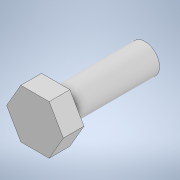
# Autodesk Inventor part: M4_short
Saved by Autodesk Inventor 2022 (Build 260153000, 153)
## iProperties
Created: 2022-02-22
Part Number: M4_short
Material: Generic
Document SubType Name: Modeling
Designer: katha
Density: 1 g/cm^3
Appearance: Default
Author: katha
Autodesk Inventor part; units mm, degrees
ref_plane "YZ Plane" through (0, 0, 0) normal (1, 0, 0) x (0, 1, 0)
ref_plane "XZ Plane" through (0, 0, 0) normal (0, 1, 0) x (-1, 0, 0)
ref_plane "XY Plane" through (0, 0, 0) normal (0, 0, 1) x (1, 0, 0)
sketch "Sketch1" plane through (0, 0, 0) normal (0, 0, 1) x (1, 0, 0)
  line L0 (0, 0) -> (3.9, 0) construction
  line L1 (0, 0) -> (1.95, 3.3775) construction
  line L2 (0, 0) -> (-1.95, 3.3775) construction
  line L3 (0, 0) -> (-3.9, 0) construction
  line L4 (0, 0) -> (-1.95, -3.3775) construction
  line L5 (0, 0) -> (1.95, -3.3775) construction
  line L6 (-1.95, 3.3775) -> (1.95, 3.3775)
  line L7 (1.95, 3.3775) -> (3.9, 0)
  line L8 (3.9, 0) -> (1.95, -3.3775)
  line L9 (1.95, -3.3775) -> (-1.95, -3.3775)
  line L10 (-1.95, -3.3775) -> (-3.9, 0)
  line L11 (-3.9, 0) -> (-1.95, 3.3775)
  dimension "d0" = 3.9
  dimension "d3" = 360
  constraints: 24 end point, 3 parallel, 2 coincident, 2 horizontal, 17 other
  measures "d0" distance of L0.start L0.end
extrude "Extrusion1" add sketch "Sketch1" along normal blind 2.85
sketch "Sketch2" plane through (0, 0, 0) normal (0, 0, -1) x (-1, 0, 0)
  circle A0 centre (0, 0) radius 2
  dimension "d7" = 4
  constraints: 1 centre point, 1 coincident
  measures "d7" diameter of A0
extrude "Extrusion2" add sketch "Sketch2" along normal blind 12.3
body "Solid1"
